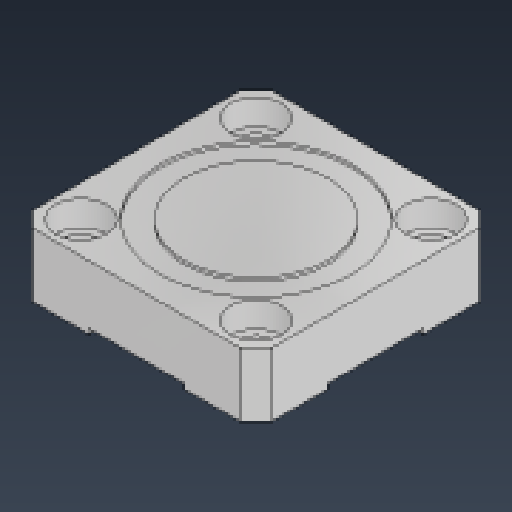
# Autodesk Inventor part: D-100.00 Capacitive Sensor
Saved by Autodesk Inventor 2025.2 (Build 292293000, 293)
## iProperties
Created: 2025-04-12
Part Number: D-100.00 Capacitive Sensor
Material: Aluminum 6061
Document SubType Name: Modeling
Designer: Kacper Mik
Density: 2.7 g/cm^3
Appearance: Aluminum - Polished
Author: Kacper Mik
Autodesk Inventor part; units mm, degrees
ref_plane "YZ Plane" through (0, 0, 0) normal (1, 0, 0) x (0, 1, 0)
ref_plane "XZ Plane" through (0, 0, 0) normal (0, 1, 0) x (-1, 0, 0)
ref_plane "XY Plane" through (0, 0, 0) normal (0, 0, 1) x (1, 0, 0)
sketch "Sketch1" plane through (0, 0, 0) normal (0, 1, 0) x (-1, 0, 0)
  line L0 (-7.5, 7.5) -> (7.5, 7.5)
  line L1 (7.5, 7.5) -> (7.5, -7.5)
  line L2 (7.5, -7.5) -> (-7.5, -7.5)
  line L3 (-7.5, -7.5) -> (-7.5, 7.5)
  line L4 (-7.5, 7.5) -> (7.5, -7.5) construction
  line L5 (7.5, 7.5) -> (-7.5, -7.5) construction
  point P0 (0, 0)
  dimension "d0" = 15
  dimension "d1" = 15
  constraints: 12 end point, 2 midpoint, 2 parallel, 1 horizontal, 1 perpendicular
  measures "d0" distance of L1.end L2.end
  measures "d1" distance of L0.end L1.end
extrude "Extrusion1" add sketch "Sketch1" along normal blind 4
sketch "Sketch2" plane through (0, 4, 0) normal (0, 1, 0) x (1, 0, 0)
  line L0 (5.5, -5.5) -> (-5.5, -5.5) construction
  line L1 (-5.5, -5.5) -> (-5.5, 5.5) construction
  line L2 (-5.5, 5.5) -> (5.5, 5.5) construction
  line L3 (5.5, 5.5) -> (5.5, -5.5) construction
  line L4 (5.5, -5.5) -> (-5.5, 5.5) construction
  line L5 (-5.5, -5.5) -> (5.5, 5.5) construction
  point P0 (0, 0)
  dimension "d4" = 11
  dimension "d5" = 11
  constraints: 12 end point, 4 coincident, 2 midpoint, 2 parallel, 1 horizontal, 1 perpendicular
  measures "d4" distance of L1.end L2.end
  measures "d5" distance of L0.end L1.end
chamfer "Chamfer1" distance 1 angle 45 4 edges at (-7.5, 2, 7.5) (7.5, 2, 7.5) (7.5, 2, -7.5) (-7.5, 2, -7.5)
hole "Hole1" at (-5.5, 4, -5.5) at (5.5, 4, -5.5) at (5.5, 4, 5.5) at (-5.5, 4, 5.5) direction (0, -1, 0) diameter 1.6 end through all counterbore diameter 3.1 counterbore depth 1.6 clearance for "Socket Head Cap Screw ISO 4762" size "M1.4" standard "ISO"
sketch "Sketch3" plane through (0, 4, 0) normal (0, 1, 0) x (1, 0, 0)
  circle A0 centre (0, 0) radius 6
  circle A1 centre (0, 0) radius 4.5
  dimension "d16" = 12
  dimension "d17" = 9
  constraints: 2 centre point, 2 coincident
  measures "d16" diameter of A0
  measures "d17" diameter of A1
extrude "Extrusion2" cut sketch "Sketch3" against normal blind 0.2
sketch "Sketch4" plane through (0, 0, 0) normal (0, -1, 0) x (1, 0, 0)
  line L0 (-6.5, 7.5) -> (6.5, 7.5) projected
  line L1 (-3, -7.5) -> (3, -7.5)
  line L2 (3, -7.5) -> (3, 7.5)
  line L3 (3, 7.5) -> (-3, 7.5)
  line L4 (-3, 7.5) -> (-3, -7.5)
  line L5 (-3, -7.5) -> (3, 7.5) construction
  line L6 (3, -7.5) -> (-3, 7.5) construction
  line L7 (7.5, 6.5) -> (7.5, -6.5) projected
  line L8 (-7.5, -3) -> (7.5, -3)
  line L9 (7.5, -3) -> (7.5, 3)
  line L10 (7.5, 3) -> (-7.5, 3)
  line L11 (-7.5, 3) -> (-7.5, -3)
  line L12 (-7.5, -3) -> (7.5, 3) construction
  line L13 (7.5, -3) -> (-7.5, 3) construction
  point P0 (0, 0)
  point P1 (-3, -3)
  point P2 (3, -3)
  point P3 (3, 3)
  point P4 (-3, 3)
  dimension "d20" = 6
  dimension "d21" = 6
  constraints: 24 end point, 4 midpoint, 4 parallel, 2 horizontal, 2 perpendicular, 2 point on line
  measures "d20" distance of L3.end L2.end
  measures "d21" distance of L9.end L8.end
extrude "Extrusion3" cut sketch "Sketch4" against normal blind 0.3
body "Solid1"
